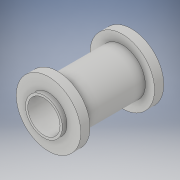
# Autodesk Inventor part: GuidingPulley
Saved by Autodesk Inventor 2019 (Build 230136000, 136)
## iProperties
Created: 2022-08-09
Part Number: GuidingPulley
Material: Generic
Document SubType Name: Modeling
Designer: zreik
Density: 1 g/cm^3
Appearance: Default
Author: zreik
Autodesk Inventor part; units mm, degrees
ref_plane "YZ Plane" through (0, 0, 0) normal (1, 0, 0) x (0, 1, 0)
ref_plane "XZ Plane" through (0, 0, 0) normal (0, 1, 0) x (-1, 0, 0)
ref_plane "XY Plane" through (0, 0, 0) normal (0, 0, 1) x (1, 0, 0)
sketch "Sketch1" plane through (0, 0, 0) normal (0, 0, 1) x (1, 0, 0)
  circle A0 centre (0, 0) radius 1.75
  circle A1 centre (0, 0) radius 3.5
  circle A2 centre (0, 0) radius 2.5
  dimension "d0" = 3.5
  dimension "d1" = 7
  dimension "d9" = 5
  constraints: 3 centre point, 3 coincident
  measures "d0" diameter of A0
  measures "d1" diameter of A1
  measures "d9" diameter of A2
extrude "Extrusion1" add sketch "Sketch1" along normal blind 9 contours A2
extrude "Extrusion2" add sketch "Sketch1" along normal blind 1 contours A1 | A2
sketch "Sketch2" plane through (0, 0, 9) normal (0, 0, 1) x (1, 0, 0)
  circle A0 centre (0, 0) radius 3.5
  circle A1 centre (0, 0) radius 1.75
  dimension "d6" = 7
  dimension "d10" = 3.5
  constraints: 2 centre point, 2 coincident
  measures "d6" diameter of A0
  measures "d10" diameter of A1
extrude "Extrusion3" add sketch "Sketch2" against normal blind 1
sketch "Sketch3" plane through (0, 0, 0) normal (0, 0, -1) x (-1, 0, 0)
  circle A0 centre (0, 0) radius 2
  circle A1 centre (0, 0) radius 1.75
  dimension "d11" = 4
  dimension "d12" = 3.5
  constraints: 2 centre point, 2 coincident
  measures "d11" diameter of A0
  measures "d12" diameter of A1
extrude "Extrusion4" add sketch "Sketch3" along normal blind 0.5
sketch "Sketch4" plane through (0, 0, 9) normal (0, 0, 1) x (1, 0, 0)
  circle A0 centre (0, 0) radius 1.75
  circle A1 centre (0, 0) radius 1.75 projected
  circle A2 centre (0, 0) radius 2
  dimension "d15" = 3.5
  dimension "d16" = 4
  constraints: 2 centre point, 2 coincident
  measures "d15" diameter of A0
  measures "d16" diameter of A2
extrude "Extrusion5" add sketch "Sketch4" along normal blind 0.5
body "Solid1"
